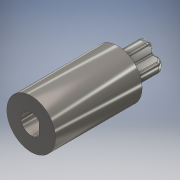
# Autodesk Inventor part: Honlite Axes Adapter
Saved by Autodesk Inventor 2016 (Build 200138000, 138)
## iProperties
Created: 2015-06-23
Part Number: Honlite Axes Adapter
Material: Generic
Document SubType Name: Modeling
Designer: 3DPrinterUser
Density: 1 g/cm^3
Appearance: Knurled 45
d66: 11,600 mm
Author: 3DPrinterUser
Autodesk Inventor part; units mm, degrees
ref_plane "XZ Plane" through (0, 0, 0) normal (0, 1, 0) x (-1, 0, 0)
ref_plane "XY Plane" through (0, 0, 0) normal (0, 0, 1) x (1, 0, 0)
sketch "Sketch1" plane through (0, 0, 0) normal (0, 1, 0) x (-1, 0, 0)
  circle A0 centre (0, 0) radius 6.75
  dimension "d0" = 13.5
  constraints: 1 centre point, 1 coincident
  measures "d0" diameter of A0
extrude "Extrusion1" add sketch "Sketch1" along normal blind 21
ref_plane "Work Plane1" through (6.75, 0, 0) normal (1, 0, 0) x (0, 1, 0)
sketch "Sketch3" plane through (0, 21, 0) normal (0, 1, 0) x (1, 0, 0)
  circle A0 centre (0, 0) radius 6.75 projected
extrude "Extrusion2" add sketch "Sketch3" along normal blind 3
sketch "Sketch4" plane through (0, 24, 0) normal (0, 1, 0) x (1, 0, 0)
  line L0 (-1.35, 4.5) -> (-1.35, 1.35)
  line L1 (-1.35, 1.35) -> (-4.5, 1.35)
  line L2 (-4.5, 1.35) -> (-4.5, -1.35)
  line L3 (-4.5, -1.35) -> (-1.35, -1.35)
  line L4 (-1.35, -1.35) -> (-1.35, -4.5)
  line L5 (1.35, -4.5) -> (1.35, -1.35)
  line L6 (1.35, -1.35) -> (4.5, -1.35)
  line L7 (4.5, -1.35) -> (4.5, 1.35)
  line L8 (4.5, 1.35) -> (1.35, 1.35)
  line L9 (1.35, 1.35) -> (1.35, 4.5)
  line L10 (0, 9.45) -> (0, -9.45) construction
  circle A0 centre (0, 0) radius 6.75 construction
  line L11 (-6.75, 0) -> (6.75, 0) construction
  line L12 (-1.35, 4.5) -> (1.35, 4.5)
  line L13 (-1.35, -4.5) -> (1.35, -4.5)
  dimension "d25" = 2.7
  dimension "d26" = 2.7
  dimension "d27" = 9
  dimension "d28" = 9
  constraints: 26 end point, 6 point on line, 4 perpendicular, 3 horizontal, 2 point on circle, 2 vertical, 1 midpoint, 1 parallel, 4 other
  measures "d25" distance between parallel lines of L9 L0
  measures "d26" distance of L1.end L2.end
  measures "d27" diameter of L12 L11
  measures "d28" distance between parallel lines of L2 L7
extrude "Extrusion3" add sketch "Sketch4" along normal blind 8.6
sketch "Sketch6" plane through (0, 0, 0) normal (1, 0, 0) x (0, 1, 0)
  line L0 (24, 1.35) -> (24, 4.5) projected
  line L1 (24, 1.35) -> (32.6, 1.35) projected
  line L2 (32.6, 4.5) -> (32.6, 1.35) projected
  line L3 (24, 4.5) -> (32.6, 4.5) projected
  line L4 (32.6, 1.35) -> (32.6, 4.5) projected
  line L5 (24, 4.5) -> (32.6, 4.5) projected
  arc A0 (32.6, 2.75) -> (30.85, 4.5) centre (30.85, 2.75) ccw
  line L6 (30.85, 4.5) -> (30.85, 7.0112)
  line L7 (30.85, 7.0112) -> (34.4134, 7.0112)
  line L8 (34.4134, 7.0112) -> (34.4134, 2.75)
  line L9 (34.4134, 2.75) -> (32.6, 2.75)
  line L10 (-6.9827, 0) -> (41.8961, 0) projected
  line L11 (30.85, 7.0112) -> (24, 7.0112)
  line L12 (24, 7.0112) -> (24, 4.5)
  line L13 (24, -6.75) -> (24, 6.75) projected
  line L14 (24, 4.5) -> (32.6, 4.5) projected
  line L15 (30.85, 4.5) -> (24, 4.5)
  point P0 (4.5, -15)
  dimension "d52" = 1.4
  constraints: 14 end point, 3 perpendicular, 2 collinear, 2 point on circle, 2 point on line, 2 tangent, 1 centre point, 1 horizontal, 1 vertical
  measures "d52" vertical distance of L1.end A0.centre
revolve "Revolution1" cut sketch "Sketch6" angle 360 about axis through (0, -10, 0) along (0, 1, 0) contours L12 L11 L6 L3 | L6 L7 L8 L9 L2 L3 | L3 L2 A0
fillet "Fillet6" radius 0.6 24 edges at (1.35, 32.115, 3.722) (1.35, 32.6, 1.8729) (1.35, 27.425, 4.2927) (-1.35, 32.6, 1.8729) (-1.35, 27.425, 4.2927) (-1.35, 32.115, 3.722) (-4.2927, 27.425, 1.35) (-1.8729, 32.6, 1.35) (-3.722, 32.115, 1.35) (-3.722, 32.115, -1.35) (-1.8729, 32.6, -1.35) (-4.2927, 27.425, -1.35) (-1.35, 27.425, -4.2927) (-1.35, 32.6, -1.8729) (-1.35, 32.115, -3.722) (1.35, 32.115, -3.722) (1.35, 32.6, -1.8729) (1.35, 27.425, -4.2927) (3.722, 32.115, -1.35) (1.8729, 32.6, -1.35) (4.2927, 27.425, -1.35) (3.722, 32.115, 1.35) (1.8729, 32.6, 1.35) (4.2927, 27.425, 1.35)
fillet "Fillet2" radius 0.4 4 edges at (1.35, 28, 1.35) (1.35, 28, -1.35) (-1.35, 28, -1.35) (-1.35, 28, 1.35)
ref_plane "Work Plane2" through (0, 25.5, 0) normal (0, 1, 0) x (1, 0, 0)
sketch "Sketch5" plane through (0, 25.5, 0) normal (0, 1, 0) x (1, 0, 0)
  circle A0 centre (0, 0) radius 2.0042
  constraints: 1 centre point, 1 coincident
sketch "Sketch7" plane through (0, 24, 0) normal (0, 1, 0) x (1, 0, 0)
  circle A0 centre (0, 0) radius 6.75 projected
loft "Loft2" add profiles "Sketch5" section 1 edges at (-6.75, 24, 0)
sketch "Sketch8" plane through (0, 0, 0) normal (1, 0, 0) x (0, 1, 0)
  line L0 (24, -6.75) -> (24, 6.75) projected
  line L1 (0, 6.75) -> (0, -6.75) projected
  line L2 (21, 0) -> (24, 0) construction
  line L3 (0, 0) -> (1.5, 0) construction
  line L4 (21, 0) -> (32.6, 0)
  line L5 (32.6, -0.75) -> (32.6, 0.75) projected
  dimension "d53" = 3
  dimension "d66" = 11.6
  constraints: 6 end point, 2 horizontal, 2 midpoint
  measures "d53" distance of L2.start L2.end
  measures "d66" distance of L2.start L4.end
hole "Hole1" at (0, 0, 0) direction (0, 1, 0) diameter 5.6 depth 21 tip angle 118
sketch "Sketch11" plane through (0, 0, 0) normal (0, -1, 0) x (1, 0, 0)
  circle A0 centre (0, 0) radius 2.8 projected
  circle A1 centre (0, 0) radius 2.8 projected
  line L0 (2.22, 1.7063) -> (2.22, -1.7063)
  dimension "d69" = 2.22
  constraints: 4 point on circle, 2 end point, 1 vertical
  measures "d69" distance from line of L0 point (0, 0)
extrude "Extrusion5" add sketch "Sketch11" against normal up to surface contours A0 L0 round surface about axis through (0, 21.8412, 0) along (0, -1, 0) radius 1.4 half angle 59 far side no picked at (2.4133, 0)
sketch "Sketch2" plane through (6.75, 0, 0) normal (1, 0, 0) x (0, 1, 0)
  line L0 (0, 6.75) -> (0, -6.75) projected
  line L1 (12, 0) -> (0, 0)
  dimension "d43" = 12
  constraints: 2 end point, 1 midpoint
  measures "d43" distance from line of L0 L1.start
hole "Hole2" [suppressed]
equation "\"d26\" = d25"
equation "\"d28\" = d27"
body "Solid1"
